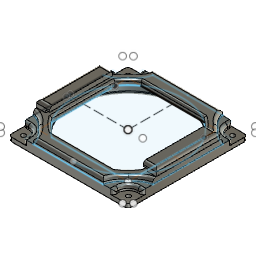
120mm fan to 100mm hepa filter adapter v4 (Autodesk Fusion 360 design; units mm, degrees)
Autodesk Fusion 360 part; units mm, degrees
note: some values were not read from the file. Chosen so that the rebuilt part matches the saved one: which face or edge a step refers to; which pieces of a blend or face edit are solid. Set by a fixed rule: which sketch regions a step uses.
sketch "Sketch1" plane through (0, 0, 0) normal (0, 0, 1) x (1, 0, 0)
  line L0 (0, 0) -> (120, 0)
  line L1 (120, 0) -> (120, 120)
  line L2 (120, 120) -> (0, 120)
  line L3 (0, 120) -> (0, 0)
  line L4 (60, 120) -> (60, 0) construction
  line L5 (0, 60) -> (120, 60) construction
  circle A0 centre (60, 60) radius 55.000002
  line L6 (0, 120) -> (7.5, 120) construction
  line L7 (7.5, 120) -> (7.5, 0) construction
  line L8 (0, 0) -> (0, 7.5) construction
  line L9 (0, 7.5) -> (120, 7.5) construction
  line L10 (0, 120) -> (0, 112.5) construction
  line L11 (0, 112.5) -> (120, 112.5) construction
  circle A1 centre (7.5, 112.5) radius 2.25
  line L12 (120, 120) -> (112.5, 120) construction
  line L13 (112.5, 120) -> (113.000002, 0) construction
  circle A2 centre (112.53125, 112.5) radius 2.25
  circle A3 centre (112.968752, 7.5) radius 2.25
  circle A4 centre (7.5, 7.5) radius 2.25
  dimension "d1" = 120
  dimension "d2" = 120
  dimension "d3" = 7.5
  dimension "d4" = 7.5
  dimension "d5" = 7.5
  dimension "d6" = 4.5
  dimension "d7" = 7.5
  dimension "d8" = 4.5
  dimension "d9" = 4.5
  dimension "d10" = 4.5
  constraint coincident L0.start L3.end
  constraint horizontal L0
  constraint perpendicular L0 L1
  constraint perpendicular L1 L2
  constraint perpendicular L0 L3
  constraint midpoint L2 L4.start
  constraint midpoint L0 L4.end
  constraint midpoint L3 L5.start
  constraint midpoint L1 L5.end
  constraint midpoint L4 A0.centre
  constraint perpendicular L3 L6
  constraint coincident L0 L7.end
  constraint perpendicular L0 L7
  constraint perpendicular L0 L8
  constraint coincident L1 L9.end
  constraint perpendicular L1 L9
  constraint perpendicular L6 L10
  constraint coincident L1 L11.end
  constraint perpendicular L1 L11
  constraint coincident L7 A1.centre
  constraint coincident L11 A1.centre
  constraint perpendicular L1 L12
  constraint coincident L7 A4.centre
  constraint coincident L9 A4.centre
  measures "d1" distance of L0.start L0.end
  measures "d2" distance of L0.end L1.end
  measures "d3" distance of L2.end L6.end
  measures "d4" distance of L0.start L8.end
  measures "d5" distance of L2.end L10.end
  measures "d6" diameter of A1
  measures "d7" distance of L1.end L12.end
  measures "d8" diameter of A2
  measures "d9" diameter of A3
  measures "d10" diameter of A4
extrude "Extrude1" add sketch "Sketch1" along normal blind 4
sketch "Sketch2" plane through (0, 0, 4) normal (0, 0, 1) x (-1, 0, 0)
  circle A0 centre (-112.53125, -112.5) radius 2.25
  circle A1 centre (-7.5, -7.5) radius 2.25
  circle A2 centre (-112.968752, -7.5) radius 2.25
  circle A3 centre (-60, -60) radius 55.000002
  circle A4 centre (-7.5, -112.5) radius 2.25
  line L0 (0, -120) -> (0, 0)
  line L1 (0, 0) -> (-120, 0)
  line L2 (-120, 0) -> (-120, -120)
  line L3 (-120, -120) -> (0, -120)
  line L4 (0, -120) -> (-120, -120)
  line L5 (-120, 0) -> (0, 0)
  line L6 (0, 0) -> (0, -120)
  line L7 (-120, -120) -> (-120, 0)
  line L8 (-120, 0) -> (-120, -5) construction
  line L9 (-120, -5) -> (-115, -5) construction
  line L10 (-120, -120) -> (-115, -120) construction
  line L11 (-120, -120) -> (-120, -115.000002) construction
  line L12 (0, -120) -> (0, -115) construction
  line L13 (0, -120) -> (-5, -120) construction
  line L14 (0, 0) -> (0, -5) construction
  line L15 (0, 0) -> (-5, 0) construction
  line L16 (-5, -59.985975) -> (-5, -60.014025)
  line L17 (-59.985817, -5) -> (-60.014183, -5)
  line L18 (-120, -120) -> (-120, 0)
  line L19 (-120, 0) -> (0, 0)
  line L20 (0, 0) -> (0, -120)
  line L21 (0, -120) -> (-120, -120)
  line L22 (-115, -5) -> (-115, -15) construction
  line L23 (-115, -5) -> (-105, -5) construction
  arc A5 (-15, -5) -> (-5, -15) centre (-5, -5) ccw
  arc A6 (-5, -105.000002) -> (-15, -115.000002) centre (-5, -115.000002) ccw
  arc A7 (-105.000002, -115.000002) -> (-115.000002, -105.000002) centre (-115.000002, -115.000002) ccw
  arc A8 (-115, -15) -> (-105, -5) centre (-115, -5) ccw
  line L24 (-115, -5) -> (-115, -8.467745) construction
  line L25 (-115.000001, -60.009707) -> (-115.000001, -59.990291)
  line L26 (-115, -8.467745) -> (-115, -5)
  line L27 (-5, -15) -> (-5, -25) construction
  line L28 (-15, -5) -> (-25, -5) construction
  line L29 (-105, -5) -> (-95, -5) construction
  line L30 (-115, -15) -> (-115, -25) construction
  line L31 (-115.000002, -105.000002) -> (-115.000001, -95.000002) construction
  line L32 (-105.000002, -115.000002) -> (-95.000002, -115.000002) construction
  line L33 (-15, -115.000002) -> (-25, -115.000002) construction
  line L34 (-5, -105.000002) -> (-5, -95.000002) construction
  line L35 (-5, -105.000002) -> (0, -105.000002)
  line L36 (-15, -115.000002) -> (-15, -120.000002)
  line L37 (-105.000002, -115.000002) -> (-105.000002, -120.000002)
  line L38 (-115.000002, -105.000002) -> (-120, -105.000001)
  line L39 (-115, -15) -> (-120.000002, -15)
  line L40 (-105, -5) -> (-105, 0)
  line L41 (-15, -5) -> (-15, 0)
  line L42 (-5, -15) -> (0, -15)
  arc A9 (-5, -60.000001) -> (-60, -5) centre (-60, -60) ccw
  arc A10 (-60, -5) -> (-115.000001, -60.000001) centre (-59.999999, -60.000002) ccw
  arc A11 (-115.000001, -60.000001) -> (-60.000001, -115.000002) centre (-60.000001, -60.000002) ccw
  arc A12 (-60.000001, -115.000002) -> (-5, -60.000001) centre (-60.000001, -60.000001) ccw
  circle A13 centre (-60.000001, -60.000001) radius 55.000003 construction
  dimension "d13" = 5
  dimension "d14" = 5
  dimension "d15" = 5
  dimension "d16" = 4.999998
  dimension "d17" = 5
  dimension "d18" = 5
  dimension "d19" = 5
  dimension "d20" = 5
  dimension "d25" = 10
  dimension "d27" = 10
  dimension "d28" = 10
  dimension "d29" = 10
  dimension "d30" = 10
  dimension "d31" = 10
  dimension "d32" = 10
  dimension "d33" = 10
  dimension "d34" = 10
  constraint coincident L0.start L3.end
  constraint coincident L2.end L3.start
  constraint coincident L1.end L2.start
  constraint coincident L0.end L1.start
  constraint perpendicular L5 L8
  constraint perpendicular L2 L9
  constraint perpendicular L2 L10
  constraint vertical L11
  constraint perpendicular L4 L12
  constraint perpendicular L12 L13
  constraint perpendicular L1 L14
  constraint perpendicular L0 L15
  constraint perpendicular L3 L16
  constraint coincident L9.end L22.start
  constraint collinear L25 L26
  constraint parallel L16 L27
  constraint parallel L17 L28
  constraint parallel L17 L29
  constraint parallel L25 L30
  constraint parallel L25 L31
  constraint perpendicular L25 L32
  constraint tangent A6 L35
  constraint perpendicular L20 L35
  constraint tangent A6 L36
  constraint perpendicular L4 L36
  constraint tangent A7 L37
  constraint perpendicular L3 L37
  constraint tangent A7 L38
  constraint tangent A8 L39
  constraint parallel L38 L39
  constraint coincident L19 L40.end
  constraint tangent A8 L40
  constraint coincident L19 L41.end
  constraint tangent A5 L41
  constraint perpendicular L19 L41
  constraint coincident L6 L42.end
  constraint tangent A5 L42
  constraint perpendicular L6 L42
  constraint tangent L17 A9
  constraint tangent L25 A10
  constraint tangent L25 A11
  constraint tangent L16 A12
  constraint coincident L17 A9.end
  constraint concentric A12 A13
  measures "d13" distance of L1.end L8.end
  measures "d14" distance of L8.end L9.end
  measures "d15" distance of L2.end L10.end
  measures "d17" distance of L0.start L12.end
  measures "d18" distance of L0.start L13.end
  measures "d19" distance of L0.end L14.end
  measures "d20" distance of L0.end L15.end
  measures "d25" radius of A8
  measures "d27" distance of A5.end L27.end
  measures "d28" distance of A5.start L28.end
  measures "d29" distance of L23.end L29.end
  measures "d30" distance of L22.end L30.end
extrude "Extrude2" add sketch "Sketch2" along normal blind 5 contours L0 L1 L2 L3 L4 L5 L6 L7 L18 L19 L20 L21 A5 A6 A7 A8 L35 L36 L37 L38 L39 L40 L41 L42 picked at (-101.673091, -102.013951)
sketch "Sketch3" plane through (0, 0, 9) normal (0, 0, 1) x (-1, 0, 0)
  circle A0 centre (-59.999999, -60.000002) radius 55.000002
  line L0 (-15, -5) -> (-15, 0)
  line L1 (-15, 0) -> (-105, 0)
  line L2 (-105, 0) -> (-105, -5)
  arc A1 (-115, -15) -> (-105, -5) centre (-115, -5) ccw
  line L3 (-115, -15) -> (-120.000002, -15)
  line L4 (-120.000002, -15) -> (-120, -105.000001)
  line L5 (-120, -105.000001) -> (-115.000002, -105.000002)
  arc A2 (-105.000002, -115.000002) -> (-115.000002, -105.000002) centre (-115.000002, -115.000002) ccw
  line L6 (-105.000002, -115.000002) -> (-105.000002, -120.000002)
  line L7 (-105.000002, -120.000002) -> (-15, -120.000002)
  line L8 (-15, -120.000002) -> (-15, -115.000002)
  arc A3 (-5, -105.000002) -> (-15, -115.000002) centre (-5, -115.000002) ccw
  line L9 (-5, -105.000002) -> (0, -105.000002)
  line L10 (0, -105.000002) -> (0, -15)
  line L11 (0, -15) -> (-5, -15)
  arc A4 (-15, -5) -> (-5, -15) centre (-5, -5) ccw
  line L12 (0, -60.000001) -> (-60, -60.000002) construction
  line L13 (-60, -60.000002) -> (-59.999999, -105.000002) construction
  line L14 (-59.999999, -105.000002) -> (-91.622777, -105.000003) construction
  line L15 (-104.999999, -105.000003) -> (-15, -105.000003) construction
  line L16 (-15, -91.622782) -> (-15, -15) construction
  line L17 (-15, -15) -> (-91.622777, -15) construction
  line L18 (-104.999999, -28.377222) -> (-104.999999, -105.000003) construction
  line L19 (-91.622777, -105.000003) -> (-28.377222, -105.000003)
  line L20 (-15, -91.622782) -> (-15, -28.377221)
  line L21 (-28.377222, -15) -> (-91.622777, -15)
  line L22 (-104.999999, -28.377222) -> (-104.999999, -91.622781)
  arc A5 (0, -62.000001) -> (0, -58.000002) centre (-74.86667, -60.000002) ccw
  arc A6 (-60.000001, -5) -> (-28.377222, -15) centre (-59.999999, -60.000002) ccw
  arc A7 (-91.622777, -15) -> (-104.999999, -28.377222) centre (-59.999999, -60.000002) ccw
  arc A8 (-28.377222, -105.000003) -> (-15, -91.622782) centre (-59.999999, -60.000002) ccw
  arc A9 (-15, -28.377221) -> (-28.377222, -15) centre (-59.999999, -60.000002) ccw construction
  arc A10 (-104.999999, -91.622781) -> (-91.622777, -105.000003) centre (-59.999999, -60.000002) ccw construction
  line L23 (-28.377222, -105.000003) -> (-91.622777, -105.000003)
  line L24 (-15, -91.622782) -> (-15, -105.000003) construction
  line L25 (-91.622777, -15) -> (-104.999999, -15) construction
  line L26 (-104.999999, -28.377222) -> (-104.999999, -15) construction
  line L27 (-104.999999, -60.000002) -> (-120.000001, -60.000002) construction
  line L28 (-15, -91.622782) -> (-15, -28.377221)
  line L29 (-28.377222, -15) -> (-91.622777, -15)
  line L30 (-104.999999, -28.377222) -> (-104.999999, -91.622781)
  line L31 (-91.622777, -105.000003) -> (-28.377222, -105.000003)
  line L32 (0, -60.000001) -> (-0.000001, -25.000001)
  line L33 (0, -60.000001) -> (0.000001, -95.000001)
  line L34 (-60, -120.000002) -> (-25, -120.000002)
  line L35 (-60, -120.000002) -> (-95, -120.000002)
  line L36 (-120.000001, -60.000002) -> (-120.000001, -95.000002)
  line L37 (-120.000001, -60.000002) -> (-120.000001, -25.000002)
  line L38 (-60, 0) -> (-95, 0)
  line L39 (-60, 0) -> (-25, 0)
  arc A11 (-25, 0) -> (-15, -15) centre (1.250005, 6.666669) ccw
  arc A12 (-104.999999, -15) -> (-95, 0) centre (-121.250006, 6.66667) ccw
  arc A13 (-95, -120.000002) -> (-104.999999, -105.000003) centre (-121.24999, -126.666663) ccw
  arc A14 (-15, -105.000003) -> (-25, -120.000002) centre (1.250003, -126.666671) ccw
  arc A15 (0.000001, -95.000001) -> (-15, -105.000003) centre (6.715036, -121.322552) ccw
  arc A16 (-15, -15) -> (-0.000001, -25.000001) centre (6.715032, 1.322546) ccw
  arc A17 (-120.000001, -25.000002) -> (-104.999999, -15) centre (-126.666675, 1.250012) ccw
  arc A18 (-104.999999, -105.000003) -> (-120.000001, -95.000002) centre (-126.666674, -121.250013) ccw
  dimension "d37" = 60
  dimension "d38" = 45
  dimension "d39" = 45
  dimension "d77" = 35
  dimension "d78" = 35
  dimension "d79" = 35
  dimension "d80" = 35
  dimension "d81" = 35
  dimension "d82" = 35
  dimension "d83" = 35
  dimension "d84" = 35
  constraint perpendicular L4 L12
  constraint concentric A0 A10
  constraint perpendicular L12 L13
  constraint perpendicular L13 L14
  constraint horizontal L15
  constraint vertical L16
  constraint horizontal L17
  constraint vertical L18
  constraint horizontal L19
  constraint vertical L20
  constraint horizontal L21
  constraint vertical L22
  constraint concentric A9 A10
  constraint concentric A6 A9
  constraint concentric A6 A10
  constraint perpendicular L15 L24
  constraint perpendicular L24 L25
  constraint perpendicular L25 L26
  constraint perpendicular L12 L32
  constraint perpendicular L12 L33
  constraint parallel L7 L34
  constraint parallel L7 L35
  constraint perpendicular L27 L36
  constraint perpendicular L27 L37
  constraint parallel L1 L38
  constraint parallel L1 L39
  constraint tangent A5 A15
  constraint tangent A5 A16
  measures "d83" distance of L38.start L38.end
  measures "d84" distance of L38.start L39.end
extrude "Extrude7" add sketch "Sketch3" along normal blind 5 contours A0 L20 A6 L28 | A0 L21 A6 L29 | A0 L19 A6 L23 L31 | A0 L22 A6 L30 | L1 L4 L7 L10 L32 L33 L34 L35 L36 L37 L38 L39 A11 A12 A13 A14 A15 A16 A17 A18 picked at (-13.824275, -68.628852) picked at (-62.24042, -11.804077) picked at (-51.592131, -106.291684) picked at (-106.29168, -51.592133) picked at (-76.113922, -2.214247)
extrude "Extrude3" add sketch "Sketch3" along normal blind 5 contours A0 L20 A6 L28 | A0 L21 A6 L29 | A0 L19 A6 L23 L31 | A0 L22 A6 L30 | L10 A5 L32 L33 picked at (-13.824275, -68.628852) picked at (-62.24042, -11.804077) picked at (-51.592131, -106.291684) picked at (-106.29168, -51.592133) picked at (0.007914, -60.888913)
sketch "Sketch9" plane through (0, 0, 14) normal (0, 0, 1) x (-1, 0, 0)
  line L0 (-28.377222, -105.000003) -> (-91.622777, -105.000003)
  arc A0 (-104.999999, -91.622781) -> (-91.622777, -105.000003) centre (-59.999999, -60.000002) ccw
  line L1 (-104.999999, -91.622781) -> (-104.999999, -28.377222)
  arc A1 (-91.622777, -15) -> (-104.999999, -28.377222) centre (-59.999999, -60.000002) ccw
  line L2 (-91.622777, -15) -> (-28.377222, -15)
  arc A2 (-15, -28.377221) -> (-28.377222, -15) centre (-59.999999, -60.000002) ccw
  line L3 (-15, -28.377221) -> (-15, -91.622782)
  arc A3 (-28.377222, -105.000003) -> (-15, -91.622782) centre (-59.999999, -60.000002) ccw
  line L4 (-95, -120.000002) -> (-25, -120.000002)
  arc A4 (-15, -105.000003) -> (-25, -120.000002) centre (1.250003, -126.666671) ccw
  arc A5 (0.000001, -95.000001) -> (-15, -105.000003) centre (6.715036, -121.322552) ccw
  line L5 (0.000001, -95.000001) -> (0, -62.000001)
  arc A6 (0, -62.000001) -> (0, -58.000002) centre (-74.86667, -60.000002) ccw
  line L6 (0, -58.000002) -> (-0.000001, -25.000001)
  arc A7 (-15, -15) -> (-0.000001, -25.000001) centre (6.715032, 1.322546) ccw
  arc A8 (-25, 0) -> (-15, -15) centre (1.250005, 6.666669) ccw
  line L7 (-25, 0) -> (-95, 0)
  arc A9 (-104.999999, -15) -> (-95, 0) centre (-121.250006, 6.66667) ccw
  arc A10 (-120.000001, -25.000002) -> (-104.999999, -15) centre (-126.666675, 1.250012) ccw
  line L8 (-120.000001, -25.000002) -> (-120.000001, -95.000002)
  arc A11 (-104.999999, -105.000003) -> (-120.000001, -95.000002) centre (-126.666674, -121.250013) ccw
  arc A12 (-95, -120.000002) -> (-104.999999, -105.000003) centre (-121.24999, -126.666663) ccw
  line L9 (-15, -91.622782) -> (0.000001, -91.622782) construction
  line L10 (-103.9488, -91.622781) -> (-120.000001, -91.622781) construction
  line L11 (-15, -28.377221) -> (-0.000001, -28.377221) construction
  line L12 (-104.999999, -28.377222) -> (-120.000001, -28.377222) construction
  line L13 (-120.000001, -91.622781) -> (-111.000001, -91.622781) construction
  line L14 (-111.000001, -91.622781) -> (-111.000001, -28.377222) construction
  line L15 (-0.000001, -28.377221) -> (-9.000001, -28.377221) construction
  line L16 (-9.000001, -28.377221) -> (-8.999999, -91.622782) construction
  line L17 (0.000001, -91.622782) -> (-9.000001, -91.622782)
  line L18 (-9.000001, -91.622782) -> (-9.000001, -28.377221)
  line L19 (-9.000001, -28.377221) -> (0.000001, -28.377221)
  line L20 (0.000001, -28.377221) -> (0.000001, -91.622782)
  line L21 (-111.000001, -91.622781) -> (-120.000001, -91.622781)
  line L22 (-120.000001, -91.622781) -> (-120.000001, -28.377222)
  line L23 (-120.000001, -28.377222) -> (-111.000001, -28.377222)
  line L24 (-111.000001, -28.377222) -> (-111.000001, -91.622781)
  dimension "d87" = 9
  dimension "d88" = 9
  constraint perpendicular L5 L9
  constraint perpendicular L8 L10
  constraint perpendicular L6 L11
  constraint perpendicular L8 L12
  constraint perpendicular L1 L13
  constraint perpendicular L12 L14
  constraint perpendicular L6 L15
  constraint perpendicular L9 L16
  constraint horizontal L17
  constraint vertical L18
  constraint horizontal L19
  constraint vertical L20
  constraint horizontal L21
  constraint vertical L22
  constraint horizontal L23
  constraint vertical L24
extrude "Extrude8" add sketch "Sketch9" along normal blind 7 contours L8 L21 L22 L23 L24 | L5 L6 L17 L18 L19 L20 picked at (-114.000001, -49.459075) picked at (-6, -59.333335)
sketch "Sketch10" plane through (9.000001, 0, 0) normal (1, 0, 0) x (0, 1, 0)
  line L0 (28.377221, 14) -> (91.622782, 14)
  line L1 (91.622782, 14) -> (91.622782, 21)
  line L2 (91.622782, 21) -> (28.377221, 21)
  line L3 (28.377221, 21) -> (28.377221, 14)
  line L4 (28.377221, 14) -> (28.377221, 16.5) construction
  line L5 (28.377221, 16.5) -> (91.622782, 16.5) construction
  line L6 (28.377221, 21) -> (91.622782, 21)
  line L7 (91.622782, 21) -> (91.622782, 16.5)
  line L8 (91.622782, 16.5) -> (28.377221, 16.5)
  line L9 (28.377221, 16.5) -> (28.377221, 21)
  line L10 (28.377221, 21) -> (91.622782, 21)
  line L11 (91.622782, 21) -> (91.622782, 16.5)
  line L12 (91.622782, 16.5) -> (28.377221, 16.5)
  line L13 (28.377221, 16.5) -> (28.377221, 21)
  line L14 (28.377221, 21) -> (28.377221, 16.5)
  line L15 (28.377221, 21) -> (91.622782, 21)
  line L16 (91.622782, 21) -> (91.622782, 16.5)
  dimension "d91" = 2.5
  constraint perpendicular L0 L4
  constraint perpendicular L1 L5
  constraint horizontal L6
  constraint vertical L7
  constraint horizontal L8
  constraint vertical L9
  constraint horizontal L10
  constraint vertical L11
  constraint horizontal L12
  constraint vertical L13
extrude "Extrude9" add sketch "Sketch10" along normal blind 4 contours L1 L2 L3 L6 L7 L8 L9 L10 L11 L12 L13 L14 L15 L16 picked at (49.459075, 18)
sketch "Sketch11" plane through (111.000001, 0, 0) normal (-1, 0, 0) x (0, -1, 0)
  line L0 (-91.622781, 14) -> (-28.377222, 14)
  line L1 (-28.377222, 14) -> (-28.377222, 21)
  line L2 (-28.377222, 21) -> (-91.622781, 21)
  line L3 (-91.622781, 21) -> (-91.622781, 14)
  line L4 (-91.622781, 14) -> (-91.622781, 16.5) construction
  line L5 (-91.622781, 16.5) -> (-28.377222, 16.5)
  line L6 (-28.377222, 16.5) -> (-28.377222, 21)
  line L7 (-28.377222, 21) -> (-91.622781, 21)
  line L8 (-91.622781, 21) -> (-91.622781, 16.5)
  dimension "d94" = 2.5
  constraint perpendicular L0 L4
  constraint horizontal L5
  constraint vertical L6
  constraint horizontal L7
  constraint vertical L8
extrude "Extrude10" add sketch "Sketch11" along normal blind 4 contours L1 L2 L3 L5 L6 L7 L8 picked at (-70.540928, 19.5)
fillet "Fillet11" radius 3 40 edges at (120.000001, 60.000002, 21) (-0.000001, 60.000001, 21) (60, 120.000002, 14) (60, 0, 14) (111.643537, 98.715307, 14) (98.715304, 111.643538, 14) (21.284695, 111.643539, 14) (8.353715, 98.719429, 14) (111.643537, 21.284696, 14) (98.715304, 8.356463, 14) (21.284695, 8.356464, 14) (8.353716, 21.280573, 14) (6.5, 28.377221, 21) (6.5, 91.622782, 21) (113.500001, 28.377222, 21) (113.500001, 91.622781, 21) (0, 120, 2) (0, 0, 2) (120, 0, 2) (120, 120, 2) (120, 105.000001, 6.5) (105.000002, 120.000002, 6.5) (117.500001, 105.000002, 9) (107.928934, 107.928934, 9) (105.000002, 117.500002, 9) (15, 120.000002, 6.5) (0, 105.000002, 6.5) (15, 117.500002, 9) (12.071068, 107.928934, 9) (2.5, 105.000002, 9) (105, 0, 6.5) (105, 2.5, 9) (107.928932, 12.071068, 9) (117.500001, 15, 9) (120.000002, 15, 6.5) (15, 0, 6.5) (0, 15, 6.5) (2.5, 15, 9) (12.071068, 12.071068, 9) (15, 2.5, 9)
fillet "Fillet12" radius 2 8 edges at (98.890872, 98.890877, 14) (104.999999, 60.000002, 14) (98.890872, 21.109127, 14) (59.999999, 15, 14) (21.109127, 21.109126, 14) (21.109127, 98.890877, 14) (59.999999, 105.000003, 14) (15, 60.000002, 14)
fillet "Fillet13" radius 3 1 edges at (8.721994, 79.888849, 0)
sketch "Sketch4" plane through (0, 0, 14) normal (0, 0, 1) x (-1, 0, 0)
  line L0 (-28.377222, -105.000003) -> (-91.622777, -105.000003)
  arc A0 (-104.999999, -91.622781) -> (-91.622777, -105.000003) centre (-59.999999, -60.000002) ccw
  line L1 (-104.999999, -91.622781) -> (-104.999999, -28.377222)
  arc A1 (-91.622777, -15) -> (-104.999999, -28.377222) centre (-59.999999, -60.000002) ccw
  line L2 (-91.622777, -15) -> (-28.377222, -15)
  arc A2 (-15, -28.377221) -> (-28.377222, -15) centre (-59.999999, -60.000002) ccw
  line L3 (-15, -28.377221) -> (-15, -91.622782)
  arc A3 (-28.377222, -105.000003) -> (-15, -91.622782) centre (-59.999999, -60.000002) ccw
  arc A4 (-15, -15) -> (-104.999999, -15) centre (-60, -74.999997) ccw
  arc A5 (-104.999999, -15) -> (-104.999999, -105.000003) centre (-45.000004, -60.000002) ccw
  arc A6 (-104.999999, -105.000003) -> (-15, -105.000003) centre (-60, -44.999999) ccw
  arc A7 (-15, -105.000003) -> (0, -62.000001) centre (-74.86667, -60.000002) ccw
  line L4 (0, -62.000001) -> (0, -58.000002)
  arc A8 (0, -58.000002) -> (-15, -15) centre (-74.86667, -60.000002) ccw
  line L5 (-59.999999, -105.000003) -> (-59.999999, -15) construction
  line L6 (-59.999999, -60.000002) -> (-106.999999, -60.000002) construction
  line L7 (-59.999999, -60.000002) -> (-12.999999, -60.000002) construction
  line L8 (-106.999999, -60.000002) -> (-106.999999, -90.000001) construction
  line L9 (-106.999999, -60.000002) -> (-106.999999, -30.000002) construction
  line L10 (-12.999999, -60.000002) -> (-12.999999, -90.000002) construction
  line L11 (-12.999999, -60.000002) -> (-12.999999, -30.000002) construction
  line L12 (-12.999999, -60.000002) -> (-7.999999, -60.000002) construction
  line L13 (-106.999999, -60.000002) -> (-111.999999, -60.000002) construction
  line L14 (-111.999999, -60.000002) -> (-111.999999, -90.000002) construction
  line L15 (-7.999999, -60.000002) -> (-7.999999, -90.000002) construction
  line L16 (-7.999999, -90.000002) -> (-12.999999, -90.000002)
  line L17 (-12.999999, -90.000002) -> (-12.999999, -30.000002)
  line L18 (-12.999999, -30.000002) -> (-7.999999, -30.000002)
  line L19 (-7.999999, -30.000002) -> (-7.999999, -90.000002)
  line L20 (-111.999999, -90.000002) -> (-106.999999, -90.000002)
  line L21 (-106.999999, -90.000002) -> (-106.999999, -30.000002)
  line L22 (-106.999999, -30.000002) -> (-111.999999, -30.000002)
  line L23 (-111.999999, -30.000002) -> (-111.999999, -90.000002)
  dimension "d42" = 47
  dimension "d43" = 47
  dimension "d44" = 30
  dimension "d45" = 30
  dimension "d46" = 30
  dimension "d47" = 5
  dimension "d48" = 5
  dimension "d49" = 30
  dimension "d50" = 30
  constraint perpendicular L5 L6
  constraint perpendicular L5 L7
  constraint perpendicular L6 L8
  constraint perpendicular L6 L9
  constraint perpendicular L7 L10
  constraint perpendicular L7 L11
  constraint perpendicular L11 L12
  constraint perpendicular L8 L13
  constraint perpendicular L13 L14
  constraint perpendicular L12 L15
  constraint horizontal L16
  constraint vertical L17
  constraint horizontal L18
  constraint vertical L19
  constraint horizontal L20
  constraint vertical L21
  constraint horizontal L22
  constraint vertical L23
sketch "Sketch8" plane through (0, 0, 14) normal (0, 0, 1) x (-1, 0, 0)
  line L0 (-28.377222, -105.000003) -> (-91.622777, -105.000003)
  arc A0 (-104.999999, -91.622781) -> (-91.622777, -105.000003) centre (-59.999999, -60.000002) ccw
  line L1 (-104.999999, -91.622781) -> (-104.999999, -28.377222)
  arc A1 (-91.622777, -15) -> (-104.999999, -28.377222) centre (-59.999999, -60.000002) ccw
  line L2 (-91.622777, -15) -> (-28.377222, -15)
  arc A2 (-15, -28.377221) -> (-28.377222, -15) centre (-59.999999, -60.000002) ccw
  line L3 (-15, -28.377221) -> (-15, -91.622782)
  arc A3 (-28.377222, -105.000003) -> (-15, -91.622782) centre (-59.999999, -60.000002) ccw
  arc A4 (-15, -15) -> (-104.999999, -15) centre (-60, -74.999997) ccw
  arc A5 (-104.999999, -15) -> (-104.999999, -105.000003) centre (-45.000004, -60.000002) ccw
  arc A6 (-104.999999, -105.000003) -> (-15, -105.000003) centre (-60, -44.999999) ccw
  arc A7 (-15, -105.000003) -> (0, -62.000001) centre (-74.86667, -60.000002) ccw
  line L4 (0, -62.000001) -> (0, -58.000002)
  arc A8 (0, -58.000002) -> (-15, -15) centre (-74.86667, -60.000002) ccw
  line L5 (-15, -91.622782) -> (-6.976921, -91.622782) construction
  line L6 (-6.976921, -91.622782) -> (-6.976921, -28.377221) construction
  line L7 (-6.976921, -28.377221) -> (-15, -28.377221) construction
  line L8 (-15, -28.377221) -> (-15, -91.622782) construction
  constraint horizontal L5
  constraint vertical L6
  constraint horizontal L7
  constraint vertical L8
extrude "Extrude4" [suppressed]
sketch "Sketch5" plane through (12.999999, 0, 0) normal (1, 0, 0) x (0, 1, 0)
  line L0 (30.000002, 14) -> (90.000002, 14)
  line L1 (90.000002, 14) -> (90.000002, 19)
  line L2 (90.000002, 19) -> (30.000002, 19)
  line L3 (30.000002, 19) -> (30.000002, 14)
  line L4 (30.000002, 19) -> (90.000002, 19)
  line L5 (90.000002, 19) -> (90.000002, 16.5)
  line L6 (90.000002, 16.5) -> (30.000002, 16.5)
  line L7 (30.000002, 16.5) -> (30.000002, 19)
  line L8 (30.000002, 19) -> (30.000002, 14) construction
  line L9 (30.000002, 19) -> (90.000002, 19) construction
  line L10 (90.000002, 16.5) -> (90.000002, 19) construction
  line L11 (30.000002, 16.5) -> (90.000002, 16.5) construction
  constraint horizontal L4
  constraint vertical L5
  constraint horizontal L6
  constraint vertical L7
extrude "Extrude5" [suppressed]
sketch "Sketch6" plane through (106.999999, 0, 0) normal (-1, 0, 0) x (0, -1, 0)
  line L0 (-90.000002, 14) -> (-30.000002, 14)
  line L1 (-30.000002, 14) -> (-30.000002, 19)
  line L2 (-30.000002, 19) -> (-90.000002, 19)
  line L3 (-90.000002, 19) -> (-90.000002, 14)
  line L4 (-90.000002, 14) -> (-90.000002, 19) construction
  line L5 (-90.000002, 16.5) -> (-30.000002, 16.5) construction
  line L6 (-30.000002, 19) -> (-30.000002, 16.5) construction
  line L7 (-30.000002, 19) -> (-90.000002, 19) construction
  line L8 (-90.000002, 19) -> (-90.000002, 16.5) construction
  line L9 (-90.000002, 16.5) -> (-30.000002, 16.5) construction
  line L10 (-30.000002, 16.5) -> (-30.000002, 19) construction
  line L11 (-90.000002, 19) -> (-30.000002, 19)
  line L12 (-30.000002, 19) -> (-30.000002, 16.5)
  line L13 (-30.000002, 16.5) -> (-90.000002, 16.5)
  line L14 (-90.000002, 16.5) -> (-90.000002, 19)
  constraint horizontal L7
  constraint vertical L8
  constraint horizontal L9
  constraint vertical L10
  constraint horizontal L11
  constraint vertical L12
  constraint horizontal L13
  constraint vertical L14
extrude "Extrude6" [suppressed]
fillet "Fillet1" [suppressed]
fillet "Fillet2" [suppressed]
fillet "Fillet3" [suppressed]
fillet "Fillet4" [suppressed]
fillet "Fillet5" [suppressed]
fillet "Fillet6" [suppressed]
fillet "Fillet7" [suppressed]
fillet "Fillet8" [suppressed]
fillet "Fillet9" [suppressed]
fillet "Fillet10" [suppressed]
sketch "Sketch7" plane through (0, 90.000002, 0) normal (0, 1, 0) x (-1, 0, 0)
  line L0 (-103.999999, 16.5) -> (-103.999999, 17)
  line L1 (-103.999999, 17) -> (-109.999999, 17)
  line L2 (-109.999999, 17) -> (-109.999999, 14)
  line L3 (-109.999999, 14) -> (-106.999999, 14)
  line L4 (-106.999999, 14) -> (-106.999999, 16.5)
  line L5 (-106.999999, 16.5) -> (-103.999999, 16.5)
equation "d42 = ( 94 / 2 ) * 1 mm"
